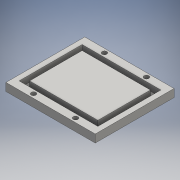
# Autodesk Inventor part: smallSampleHolder
Saved by Autodesk Inventor 2016 (Build 200138000, 138)
## iProperties
Created: 2016-04-09
Part Number: smallSampleHolder
Material: Generic
Document SubType Name: Modeling
Designer: sims01
Density: 1 g/cm^3
Appearance: Default
Author: sims01
Autodesk Inventor part; units mm, degrees
ref_plane "YZ Plane" through (0, 0, 0) normal (1, 0, 0) x (0, 1, 0)
ref_plane "XZ Plane" through (0, 0, 0) normal (0, 1, 0) x (-1, 0, 0)
ref_plane "XY Plane" through (0, 0, 0) normal (0, 0, 1) x (1, 0, 0)
sketch "Sketch1" plane through (0, 0, 0) normal (0, 0, 1) x (1, 0, 0)
  line L0 (-42.5, 37.5) -> (42.5, 37.5)
  line L1 (42.5, 37.5) -> (42.5, -37.5)
  line L2 (42.5, -37.5) -> (-42.5, -37.5)
  line L3 (-42.5, -37.5) -> (-42.5, 37.5)
  point P0 (0, 0)
  dimension "d0" = 85
  dimension "d1" = 75
  dimension "d2" = 37.5
  dimension "d3" = 42.5
  constraints: 8 end point, 2 parallel, 1 horizontal, 1 perpendicular
  measures "d0" distance of L0.start L0.end
  measures "d1" distance of L2.end L0.start
  measures "d2" distance from line of point (0, 0) L0
  measures "d3" distance from line of point (0, 0) L1
extrude "Extrusion1" add sketch "Sketch1" along normal blind 7.5
sketch "Sketch2" plane through (0, 0, 7.5) normal (0, 0, 1) x (1, 0, 0)
  point P0 (0, 0)
  point P1 (20, -33.75)
  point P2 (-20, -33.75)
  point P3 (-20, 33.75)
  point P4 (20, 33.75)
  dimension "d6" = 40
  dimension "d7" = 20
  dimension "d8" = 67.5
  dimension "d9" = 33.75
  constraints: 2 horizontal alignment, 2 vertical alignment
  measures "d6" distance of point (20, -33.75) point (-20, -33.75)
  measures "d7" horizontal distance of point (0, 0) point (-20, -33.75)
  measures "d8" distance of point (-20, 33.75) point (-20, -33.75)
  measures "d9" vertical distance of point (0, 0) point (-20, 33.75)
hole "Hole1" at (20, -33.75, 7.5) at (-20, -33.75, 7.5) at (-20, 33.75, 7.5) at (20, 33.75, 7.5) direction (0, 0, -1) diameter 4.5 depth 9.525 tip angle 118 clearance for "Countersunk Flat Head Screw ISO 2009/7046" size "M4" standard "ISO"
sketch "Sketch3" plane through (0, 0, 7.5) normal (0, 0, 1) x (1, 0, 0)
  line L0 (-37.5, -30) -> (37.5, -30)
  line L1 (37.5, -30) -> (37.5, 30)
  line L2 (37.5, 30) -> (-37.5, 30)
  line L3 (-37.5, 30) -> (-37.5, -30)
  line L4 (-32.5, -25) -> (32.5, -25)
  line L5 (32.5, -25) -> (32.5, 25)
  line L6 (32.5, 25) -> (-32.5, 25)
  line L7 (-32.5, 25) -> (-32.5, -25)
  point P0 (0, 0)
  dimension "d19" = 75
  dimension "d22" = 60
  dimension "d23" = 30
  dimension "d24" = 5
  dimension "d26" = 37.5
  dimension "d27" = 5
  dimension "d29" = 5
  dimension "d30" = 5
  constraints: 16 end point, 4 parallel, 2 horizontal, 2 perpendicular
  measures "d19" distance of L1.end L2.end
  measures "d22" distance of L2.end L0.start
  measures "d23" distance from line of point (0, 0) L0
  measures "d24" distance between parallel lines of L1 L5
  measures "d26" distance from line of L3 point (0, 0)
  measures "d27" distance between parallel lines of L7 L3
  measures "d29" distance between parallel lines of L0 L4
  measures "d30" distance between parallel lines of L2 L6
extrude "Extrusion2" cut sketch "Sketch3" against normal blind 6
equation "\"d2\" = 0.5 * d1"
equation "\"d3\" = 0.5 * d0"
equation "\"d7\" = 0.5 * d6"
equation "\"d9\" = 0.5 * d8"
equation "\"d23\" = 0.5 * d22"
equation "\"d26\" = 0.5 * d19"
equation "\"d27\" = d24"
equation "\"d29\" = d24"
equation "\"d30\" = d24"
body "Solid1"
